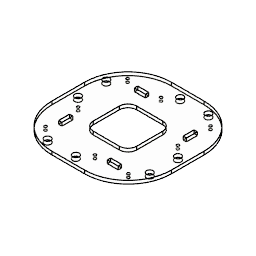
MidPlate_v8 (Autodesk Fusion 360 design; units mm, degrees)
Autodesk Fusion 360 part; units mm, degrees
sketch "Sketch1" plane through (0, 0, 0) normal (0, 0, 1) x (1, 0, 0)
  line L0 (-33.4, -17.4) -> (-33.4, 33.4) construction
  line L1 (-33.4, 33.4) -> (-27.4, 33.4) construction
  line L2 (-33.4, -17.4) -> (-36.4, -17.4)
  line L3 (-36.4, -17.4) -> (-36.4, -27.4)
  line L4 (-36.4, -27.4) -> (-33.4, -27.4)
  line L5 (-33.4, -27.4) -> (-33.4, -17.4)
  line L6 (-27.4, 33.4) -> (-17.4, 33.4)
  line L7 (-17.4, 33.4) -> (-17.4, 36.4)
  line L8 (-17.4, 36.4) -> (-27.4, 36.4)
  line L9 (-27.4, 36.4) -> (-27.4, 33.4)
  line L10 (-17.4, 33.4) -> (33.4, 33.4) construction
  line L11 (33.4, 33.4) -> (33.4, 27.4) construction
  line L12 (33.4, 27.4) -> (36.4, 27.4)
  line L13 (36.4, 27.4) -> (36.4, 17.4)
  line L14 (36.4, 17.4) -> (33.4, 17.4)
  line L15 (33.4, 17.4) -> (33.4, 27.4)
  line L16 (33.4, 17.4) -> (33.4, -33.4) construction
  line L17 (33.4, -33.4) -> (27.4, -33.4) construction
  line L18 (27.4, -33.4) -> (17.4, -33.4)
  line L19 (17.4, -33.4) -> (17.4, -36.4)
  line L20 (17.4, -36.4) -> (27.4, -36.4)
  line L21 (27.4, -36.4) -> (27.4, -33.4)
  line L22 (17.4, -33.4) -> (-33.4, -33.4) construction
  line L23 (-33.4, -33.4) -> (-33.4, -27.4) construction
  line L24 (33.4, 33.4) -> (-33.4, -33.4) construction
  line L25 (33.4, -33.4) -> (-33.4, 33.4) construction
  line L26 (55, -55) -> (-55, -55)
  line L27 (-55, -55) -> (-55, 55)
  line L28 (-55, 55) -> (55, 55)
  line L29 (55, 55) -> (55, -55)
  line L30 (55, -55) -> (-55, 55) construction
  line L31 (-55, -55) -> (55, 55) construction
  line L32 (-34.9, -17.4) -> (-34.9, -7.75) construction
  line L33 (-34.9, -7.75) -> (-38.15, -7.75) construction
  circle A0 centre (-38.15, -7.75) radius 1.25
  line L34 (-34.9, -27.4) -> (-34.9, -38.15) construction
  line L35 (-34.9, -38.15) -> (-37.75, -38.15) construction
  circle A1 centre (-37.75, -38.15) radius 1.25
  circle A2 centre (38.15, -37.75) radius 1.25
  circle A3 centre (7.75, -38.15) radius 1.25
  circle A4 centre (37.75, 38.15) radius 1.25
  circle A5 centre (38.15, 7.75) radius 1.25
  circle A6 centre (-38.15, 37.75) radius 1.25
  circle A7 centre (-7.75, 38.15) radius 1.25
  constraint vertical L0
  constraint perpendicular L0 L1
  constraint horizontal L2
  constraint vertical L3
  constraint horizontal L4
  constraint vertical L5
  constraint horizontal L6
  constraint vertical L7
  constraint horizontal L8
  constraint vertical L9
  constraint perpendicular L7 L10
  constraint perpendicular L10 L11
  constraint horizontal L12
  constraint vertical L13
  constraint horizontal L14
  constraint vertical L15
  constraint perpendicular L14 L16
  constraint perpendicular L16 L17
  constraint horizontal L18
  constraint vertical L19
  constraint horizontal L20
  constraint vertical L21
  constraint perpendicular L19 L22
  constraint coincident origin L24
  constraint coincident origin L25
  constraint horizontal L26
  constraint perpendicular L26 L27
  constraint parallel L26 L28
  constraint parallel L27 L29
  constraint coincident L30 origin
  constraint coincident L31 origin
  constraint midpoint L2 L32.start
  constraint perpendicular L2 L32
  constraint perpendicular L32 L33
  constraint coincident L33.end A0.centre
  constraint midpoint L4 L34.start
  constraint perpendicular L4 L34
  constraint perpendicular L34 L35
  constraint coincident L35.end A1.centre
  measures "d1" distance of L0.start L0.end
  measures "d2" distance of L0.end L1.end
  measures "d3" distance of L0.start L2.end
  measures "d4" distance of L0.start L4.end
  measures "d5" distance of L1.end L6.end
  measures "d6" distance of L1.end L8.end
  measures "d7" distance of L6.end L10.end
  measures "d8" distance of L10.end L11.end
  measures "d9" distance of L11.end L12.end
  measures "d10" distance of L11.end L14.end
  measures "d11" distance of L14.end L16.end
  measures "d12" distance of L16.end L17.end
  measures "d13" distance of L17.end L18.end
  measures "d14" distance of L17.end L20.end
  measures "d15" distance of L18.end L22.end
  measures "d16" distance of L27.end L28.end
  measures "d17" distance of L26.end L27.end
  measures "d22" distance of L32.start L32.end
  measures "d23" distance of L32.end L33.end
  measures "d24" diameter of A0
  measures "d25" distance of L34.start L34.end
  measures "d26" distance of L34.end L35.end
  measures "d27" diameter of A1
extrude "Extrude1" add sketch "Sketch1" along normal blind 3 contours L26 L27 L28 L29 | A0 | A1 | A2 | A3 | A4 | A5 | A6 | A7
extrude "Extrude2" cut sketch "Sketch1" along normal blind 3 contours A0 | A1 | A2 | A3 | A4 | A5 | A6 | A7
fillet "Fillet1" radius 40 4 edges at (-55, 55, 1.5) (55, 55, 1.5) (55, -55, 1.5) (-55, -55, 1.5)
derive "Sketch1 (1)" from "BasePlate v7"
sketch "Sketch2" plane through (0, 0, 0) normal (0, 0, -1) x (1, 0, 0)
  circle A0 centre (7.75, 38.15) radius 1.25
  circle A1 centre (-7.75, -38.15) radius 1.25
  circle A2 centre (37.75, -38.15) radius 1.25
  circle A3 centre (-37.75, 38.15) radius 1.25
  circle A4 centre (38.15, 37.75) radius 1.25
  circle A5 centre (-38.15, -37.75) radius 1.25
  circle A6 centre (38.15, -7.75) radius 1.25
  circle A7 centre (-38.15, 7.75) radius 1.25
  line L0 (33.4, -17.4) -> (36.4, -17.4)
  line L1 (36.4, -17.4) -> (36.4, -27.4)
  line L2 (36.4, -27.4) -> (33.4, -27.4)
  line L3 (33.4, -27.4) -> (33.4, -17.4)
  line L4 (27.4, 36.4) -> (27.4, 33.4)
  line L5 (27.4, 33.4) -> (17.4, 33.4)
  line L6 (17.4, 33.4) -> (17.4, 36.4)
  line L7 (17.4, 36.4) -> (27.4, 36.4)
  line L8 (-33.4, 27.4) -> (-33.4, 17.4)
  line L9 (-33.4, 17.4) -> (-36.4, 17.4)
  line L10 (-36.4, 17.4) -> (-36.4, 27.4)
  line L11 (-36.4, 27.4) -> (-33.4, 27.4)
  line L12 (-27.4, -36.4) -> (-27.4, -33.4)
  line L13 (-27.4, -33.4) -> (-17.4, -33.4)
  line L14 (-17.4, -33.4) -> (-17.4, -36.4)
  line L15 (-17.4, -36.4) -> (-27.4, -36.4)
  arc A8 (-15, 55) -> (-55, 15) centre (-15, 15) ccw
  line L16 (-55, 15) -> (-55, -15)
  arc A9 (-55, -15) -> (-15, -55) centre (-15, -15) ccw
  line L17 (-15, -55) -> (15, -55)
  arc A10 (15, -55) -> (55, -15) centre (15, -15) ccw
  line L18 (55, -15) -> (55, 15)
  arc A11 (55, 15) -> (15, 55) centre (15, 15) ccw
  line L19 (15, 55) -> (-15, 55)
  circle A12 centre (-27, 47) radius 3
  circle A13 centre (-1, 47) radius 3
  line L20 (-1, 47) -> (-27, 47) construction
  circle A14 centre (-47, -27) radius 3
  circle A15 centre (-47, -1) radius 3
  line L21 (-47, -1) -> (-47, -27) construction
  circle A16 centre (27, -47) radius 3
  circle A17 centre (1, -47) radius 3
  line L22 (1, -47) -> (27, -47) construction
  circle A18 centre (47, 27) radius 3
  circle A19 centre (47, 1) radius 3
  line L23 (47, 1) -> (47, 27) construction
  dimension "d36" = 6
  dimension "d37" = 6
  dimension "d39" = 360
  constraint coincident A13.centre L20.start
  constraint coincident A12.centre L20.end
  constraint horizontal L20
  measures "d36" diameter of A12
  measures "d37" diameter of A13
extrude "Extrude4" cut sketch "Sketch2" against normal blind 20 contours A12 | A13 | A14 | A15 | A16 | A17 | A18 | A19
derive "Sketch1 (2)" from "TopPlate v20"
sketch "sketch 1730" plane through (0, 0, 0) normal (0, 0, 1) x (1, 0, 0)
  line L0 (55, -55) -> (-55, -55)
  line L1 (-55, -55) -> (-55, 55)
  line L2 (-55, 55) -> (55, 55)
  line L3 (55, 55) -> (55, -55)
  circle A0 centre (0, 9) radius 2
  circle A1 centre (0, -11) radius 1
  circle A2 centre (0, 0) radius 0.5
  circle A3 centre (-27, 47) radius 3
  circle A4 centre (-1, 47) radius 3
  circle A5 centre (46.8686, 27.2241) radius 3
  line L4 (46.9988, 1) -> (46.9855, 27.035) construction
  line L5 (-1, 47) -> (-27, 47) construction
  circle A6 centre (47.0008, 0.9939) radius 3
  circle A7 centre (-47, -1) radius 3
  line L6 (-47.008, -2.9175) -> (-47.0012, -29) construction
  circle A8 centre (-47, -27) radius 3
  circle A9 centre (0.0158, -47.1318) radius 3
  line L7 (1, -47) -> (27, -47) construction
  circle A10 centre (27.9746, -46.6245) radius 3
  line L8 (27.9746, -46.6245) -> (11, 0) construction
  line L9 (0, 0) -> (5, 0) construction
  line L10 (9.1207, -0.6842) -> (12.8793, 0.6842) construction
  line L11 (12.8793, 0.6842) -> (16.9846, -10.5917)
  line L12 (9.1207, -0.6842) -> (13.2259, -11.9602)
  line L13 (16.9846, -10.5917) -> (13.2259, -11.9602)
  circle A11 centre (11, 0) radius 2
  line L14 (-0.6842, -9.1207) -> (-11.9602, -13.2259)
  line L15 (-10.5917, -16.9846) -> (-11.9602, -13.2259)
  line L16 (0.6842, -12.8793) -> (-10.5917, -16.9846)
  circle A12 centre (0, -11) radius 2
  line L17 (-46.6245, -27.9746) -> (0, -11) construction
  circle A13 centre (7.7782, 7.7782) radius 2
  line L18 (7.7782, 7.7782) -> (46.8686, 27.2241) construction
  line L19 (7.7782, 7.7782) -> (8.669, 5.9875) construction
  line L20 (8.669, 5.9875) -> (19.413, 11.3322)
  line L21 (19.413, 11.3322) -> (17.6314, 14.9136)
  line L22 (17.6314, 14.9136) -> (6.8874, 9.5688)
  circle A14 centre (-7.7782, 7.7782) radius 2
  line L23 (-7.7782, 7.7782) -> (-27, 47) construction
  line L24 (-7.7782, 7.7782) -> (-9.5741, 6.898) construction
  line L25 (-9.5741, 6.898) -> (-14.855, 17.6736)
  line L26 (-5.9823, 8.6583) -> (-11.2631, 19.4339)
  line L27 (-11.2631, 19.4339) -> (-14.855, 17.6736)
  line L28 (46.9988, 1) -> (-6.364, -6.364) construction
  line L29 (0.0158, -47.1318) -> (-11, 0) construction
  line L30 (0, 9) -> (-47.008, -2.9175) construction
  circle A15 centre (7.7782, -7.7782) radius 2
  line L31 (7.7782, -7.7782) -> (-1, 47) construction
  line L32 (0, 0) -> (9, 0) construction
  circle A16 centre (-6.364, -6.364) radius 2
  line L33 (0, -11) -> (0.6842, -12.8793)
  circle A17 centre (-11, 0) radius 2
  line L34 (-11, 0) -> (-9.0525, 0.4552) construction
  line L35 (-9.0525, 0.4552) -> (-6.3214, -11.2299)
  line L36 (-6.3214, -11.2299) -> (-10.2164, -12.1403)
  line L37 (-10.2164, -12.1403) -> (-12.9475, -0.4552)
  line L38 (-6.364, -6.364) -> (-6.0906, -8.3452) construction
  line L39 (-6.0906, -8.3452) -> (5.7968, -6.7048)
  line L40 (5.7968, -6.7048) -> (5.25, -2.7423)
  line L41 (5.25, -2.7423) -> (-6.6374, -4.3827)
  line L42 (7.7782, -7.7782) -> (9.753, -7.4617) construction
  line L43 (9.753, -7.4617) -> (7.8542, 4.3871)
  line L44 (7.8542, 4.3871) -> (3.9046, 3.7542)
  line L45 (3.9046, 3.7542) -> (5.8034, -8.0946)
  line L46 (0, 9) -> (0.4915, 7.0613) construction
  line L47 (0.4915, 7.0613) -> (-11.1405, 4.1124)
  line L48 (-11.1405, 4.1124) -> (-12.1235, 7.9897)
  line L49 (-12.1235, 7.9897) -> (-0.4915, 10.9387)
  line L50 (20, -20) -> (-20, -20)
  line L51 (-20, -20) -> (-20, 20)
  line L52 (-20, 20) -> (20, 20)
  line L53 (20, 20) -> (20, -20)
  line L54 (20, -20) -> (-20, 20) construction
  line L55 (-20, -20) -> (20, 20) construction
  line L56 (15.1052, -11.276) -> (11, 0) construction
  line L57 (13.0526, -5.638) -> (14.9319, -4.9538) construction
  line L58 (13.0526, -5.638) -> (11.1733, -6.3222) construction
  line L59 (14.9319, -4.9538) -> (17.2811, -4.0985) construction
  line L60 (16.7679, -2.689) -> (17.7943, -5.508)
  line L61 (17.7943, -5.508) -> (9.3373, -8.5869)
  line L62 (16.7679, -2.689) -> (8.311, -5.7679)
  line L63 (8.311, -5.7679) -> (9.3373, -8.5869)
  line L64 (18.5222, 13.1229) -> (7.7782, 7.7782) construction
  line L65 (13.1502, 10.4505) -> (14.041, 8.6599) construction
  line L66 (14.041, 8.6599) -> (15.1545, 6.4215) construction
  line L67 (13.8115, 5.7534) -> (16.4975, 7.0896)
  line L68 (13.8115, 5.7534) -> (9.8029, 13.8115)
  line L69 (9.8029, 13.8115) -> (12.4889, 15.1476)
  line L70 (12.4889, 15.1476) -> (16.4975, 7.0896)
  line L71 (-13.0591, 18.5537) -> (-7.7782, 7.7782) construction
  line L72 (-10.4186, 13.1659) -> (-6.3778, 15.1463) construction
  line L73 (-7.0379, 16.4932) -> (-5.7177, 13.7993)
  line L74 (-7.0379, 16.4932) -> (-5.7177, 13.7993) construction
  line L75 (-5.7177, 13.7993) -> (-13.7993, 9.8387)
  line L76 (-13.7993, 9.8387) -> (-15.1196, 12.5326)
  line L77 (-15.1196, 12.5326) -> (-7.0379, 16.4932)
  line L78 (0, 9) -> (-11.632, 6.051) construction
  line L79 (-5.816, 7.5255) -> (-4.7101, 3.1635) construction
  line L80 (-6.1642, 2.7949) -> (-3.2561, 3.5321) construction
  line L81 (-3.2561, 3.5321) -> (-6.1642, 2.7949)
  line L82 (-6.1642, 2.7949) -> (-8.3759, 11.5189)
  line L83 (-8.3759, 11.5189) -> (-5.4679, 12.2561)
  line L84 (-5.4679, 12.2561) -> (-3.2561, 3.5321)
  line L85 (-11, 0) -> (-8.2689, -11.6851) construction
  line L86 (-9.6345, -5.8425) -> (-14.0164, -6.8667) construction
  line L87 (-14.3578, -5.4061) -> (-13.675, -8.3273) construction
  line L88 (-14.3578, -5.4061) -> (-13.675, -8.3273)
  line L89 (-13.675, -8.3273) -> (-4.9112, -6.279)
  line L90 (-4.9112, -6.279) -> (-5.5939, -3.3578)
  line L91 (-5.5939, -3.3578) -> (-14.3578, -5.4061)
  line L92 (5.5234, -4.7235) -> (-6.364, -6.364) construction
  line L93 (-0.4203, -5.5437) -> (-1.0354, -1.086) construction
  line L94 (-2.5214, -1.291) -> (0.4505, -0.8809) construction
  line L95 (-2.5214, -1.291) -> (0.4505, -0.8809)
  line L96 (0.4505, -0.8809) -> (1.6808, -9.7965)
  line L97 (1.6808, -9.7965) -> (-1.291, -10.2066)
  line L98 (-1.291, -10.2066) -> (-2.5214, -1.291)
  line L99 (0, -11) -> (-11.276, -15.1052) construction
  line L100 (-5.638, -13.0526) -> (-4.0985, -17.2811) construction
  line L101 (-5.508, -17.7943) -> (-2.689, -16.7679) construction
  line L102 (-2.689, -16.7679) -> (-5.508, -17.7943)
  line L103 (-5.508, -17.7943) -> (-8.5869, -9.3373)
  line L104 (-8.5869, -9.3373) -> (-5.7679, -8.311)
  line L105 (-5.7679, -8.311) -> (-2.689, -16.7679)
  line L106 (7.7782, -7.7782) -> (5.8794, 4.0707) construction
  line L107 (6.8288, -1.8538) -> (11.2721, -1.1417) construction
  line L108 (11.0348, 0.3394) -> (11.5094, -2.6228) construction
  line L109 (11.0348, 0.3394) -> (11.5094, -2.6228)
  line L110 (11.5094, -2.6228) -> (2.6228, -4.0469)
  line L111 (2.6228, -4.0469) -> (2.1481, -1.0847)
  line L112 (2.1481, -1.0847) -> (11.0348, 0.3394)
extrude "Extrude5" cut sketch "sketch 1730" along normal blind 10 contours A0 | A0 L47 L49 L84 | A14 L26 L47 L49 L82 L84 | L26 L49 L83 L84 | L47 L81 L82 L84 | A14 L26 L49 L82 L83 | A14 L26 L49 | A14 L25 L47 L48 L49 L82 | A14 L49 L82 | A14 L25 L26 L49 L75 L82 L83 | A14 L49 L82 | A14 L49 L82 | L25 L26 L75 L77 | L26 L73 L75 L77 | A14 L49 L82 | A14 L25 L49 | L25 L26 L27 L77 | L25 L75 L76 L77 | A1 L97 | A1 A12 L33 L97 | A1 L97 | A1 A12 L97 L98 | A1 A12 L33 L97 L98 | L14 A12 L39 L96 L97 L98 | L14 L16 A12 L98 L105 | L14 A12 L98 | L16 L102 L103 L105 | L14 L16 L35 L36 L103 L105 | L14 A16 L35 L39 L98 L104 L105 | L39 L41 L45 L96 L110 L111 | L39 L41 L96 L98 | L14 L15 L16 L103 | L14 L35 L104 L105 | A16 L39 L41 L90 L98 | L39 L40 L45 L110 | A15 L39 L40 L43 L45 L62 L63 L110 | L41 L95 L96 L98 | L14 L36 L103 | L14 L35 L36 | L14 L35 L36 L103 L104 | A16 L35 L89 L90 | L41 L45 L110 L111 | L40 L41 L45 L110 | A15 L61 L63 | L41 L45 L111 L112 | A16 L35 L36 L37 L89 L103 L104 | A16 L35 L89 | A16 L41 L90 | A16 L35 L41 L90 L91 | L40 L41 L43 L45 L110 L112 | A15 L43 L62 L63 | A15 L61 L63 | L12 A15 L43 L61 L62 | A16 L35 L89 L90 | A16 L35 L37 L89 L91 | A16 L35 L89 | L12 L43 L62 L110 | L12 A11 L43 L110 L112 | L43 L44 L45 L112 | L11 L12 L13 L61 | L11 L12 L61 L62 | L37 L88 L89 L91 | A17 L35 L37 L91 | L11 L12 A11 L62 L109 L110 | L12 A11 L109 L110 | L11 L60 L61 L62 | A17 | A11 L109 L112 | A11 L109 L112 | A2 | A13 | A13 L20 L22 L68 | L22 L68 L69 L70 | L20 L22 L68 L70 | L20 L67 L68 L70 | L20 L21 L22 L70 | L50 L51 L52 L53
fillet "Fillet2" radius 8 4 edges at (-20, 20, 1.5) (20, 20, 1.5) (-20, -20, 1.5) (20, -20, 1.5)
